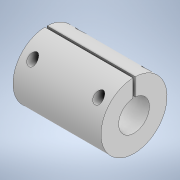
# Autodesk Inventor part: 14mm_shaft_coupler
Saved by Autodesk Inventor 2021.3 (Build 253353000, 353)
## iProperties
Created: 2023-04-09
Part Number: 14mm_shaft_coupler
Material: Generic
Document SubType Name: Modeling
Designer: nxf77172
Density: 1 g/cm^3
Appearance: Default
Author: nxf77172
Autodesk Inventor part; units mm, degrees
ref_plane "YZ Plane" through (0, 0, 0) normal (1, 0, 0) x (0, 1, 0)
sketch "Sketch1" plane through (0, 0, 0) normal (1, 0, 0) x (0, 1, 0)
  circle A0 centre (0, 0) radius 7
  circle A1 centre (0, 0) radius 15
  dimension "d0" = 14
  dimension "d1" = 30
  constraints: 3 coincident, 2 centre point
  measures "d0" diameter of A0
  measures "d1" diameter of A1
extrude "Extrusion1" add sketch "Sketch1" along normal blind 20 and the other way blind 20
ref_plane "Work Plane1" through (0, 15, 0) normal (0, 1, 0) x (-1, 0, 0)
sketch "Sketch3" plane through (0, 15, 0) normal (0, 1, 0) x (-1, 0, 0)
  line L0 (-20, 0) -> (20, 0) construction
  line L1 (-20, 15) -> (-20, -15) projected
  line L2 (20, 7) -> (20, -7) projected
  line L3 (-20, 0.5) -> (20, 0.5)
  line L4 (20, 0.5) -> (20, -0.5)
  line L5 (20, -0.5) -> (-20, -0.5)
  line L6 (-20, -0.5) -> (-20, 0.5)
  point P0 (0, 0)
  dimension "d10" = 0.5
  dimension "d11" = 0.5
  constraints: 10 end point, 2 horizontal, 2 parallel, 2 point on line, 1 midpoint, 1 perpendicular
  measures "d10" distance between parallel lines of L0 L3
  measures "d11" distance between parallel lines of L5 L0
extrude "Extrusion2" cut sketch "Sketch3" against normal up to next
ref_plane "Work Plane2" through (0, 0, -15) normal (0, 0, 1) x (1, 0, 0)
sketch "Sketch4" plane through (0, 0, -15) normal (0, 0, 1) x (1, 0, 0)
  line L0 (-20, -7) -> (-20, 6.9821) construction
  line L1 (-20, 0) -> (20, 0) construction
  line L2 (20, 6.9821) -> (20, -7) construction
  circle A0 centre (-15, 10) radius 2
  line L3 (-20, 14.9917) -> (20, 14.9917) construction
  line L4 (0, 14.9917) -> (0, -15) construction
  line L5 (-20, -15) -> (20, -15) construction
  circle A1 centre (15, 10) radius 2
  point P0 (0, 0)
  dimension "d14" = 10
  dimension "d15" = 15
  dimension "d16" = 4
  constraints: 4 end point, 3 midpoint, 2 centre point, 2 point on line, 1 horizontal, 1 symmetric about line, 1 other
  measures "d14" distance from line of A0.centre L1
  measures "d15" horizontal distance of A0.centre point (0, 0)
  measures "d16" diameter of A0
extrude "Extrusion3" cut sketch "Sketch4" along normal through all
body "Solid1"
